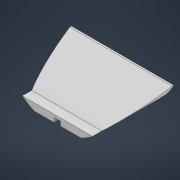
# Autodesk Inventor part: SlopeFloor
Saved by Autodesk Inventor 2021 (Build 250183000, 183)
## iProperties
Created: 2021-01-31
Part Number: SlopeFloor
Material: Generic
Document SubType Name: Modeling
Designer: argon
Density: 1 g/cm^3
Appearance: Light Gray
Author: argon
Autodesk Inventor part; units mm, degrees
ref_plane "YZ Plane" through (0, 0, 0) normal (1, 0, 0) x (0, 1, 0)
ref_plane "XZ Plane" through (0, 0, 0) normal (0, 1, 0) x (-1, 0, 0)
ref_plane "XY Plane" through (0, 0, 0) normal (0, 0, 1) x (1, 0, 0)
sketch "Sketch1" plane through (0, 0, 0) normal (0, 0, 1) x (1, 0, 0)
  circle A0 centre (0, 0) radius 1750
  line L0 (-1569.0363, -775) -> (1569.0363, -775)
  line L1 (-64, -1498) -> (64, -1498)
  line L2 (64, -1498) -> (64, -1600)
  line L3 (64, -1600) -> (-64, -1600)
  line L4 (-64, -1600) -> (-64, -1498)
  line L5 (-64, -1498) -> (64, -1600) construction
  line L6 (64, -1498) -> (-64, -1600) construction
  line L7 (97, -1633) -> (97, -1465)
  line L8 (97, -1465) -> (-97, -1465)
  line L9 (-97, -1465) -> (-97, -1633)
  line L10 (-97, -1633) -> (97, -1465) construction
  line L11 (97, -1633) -> (-97, -1465) construction
  line L12 (-708.8723, -1600) -> (708.8723, -1600)
  point P0 (0, -1549)
  point P1 (0, -1549)
  point P2 (97, -1600)
  point P3 (-97, -1600)
  dimension "d10" = 3500
  dimension "d12" = 33
  dimension "d13" = 33
  dimension "d14" = 102
  dimension "d15" = 128
  dimension "d16" = 1600
  dimension "d17" = 825
  constraints: 26 end point, 5 midpoint, 4 point on circle, 3 horizontal, 3 parallel, 1 centre point, 1 coincident, 1 collinear, 1 perpendicular, 1 vertical alignment
  measures "d10" diameter of A0
  measures "d12" distance between parallel lines of L2 L7
  measures "d13" distance between parallel lines of L1 L8
  measures "d14" distance of L2.start L2.end
  measures "d15" distance of L4.end L2.start
  measures "d16" distance from line of L3 point (0, 0)
  measures "d17" distance between parallel lines of L12 L0
extrude "Extrusion1" add sketch "Sketch1" along normal blind 2000 contours L0 A0 L12 L7 L8 L9
sketch "Sketch3" plane through (0, 0, 2000) normal (0, 0, 1) x (1, 0, 0)
  arc A0 (-1569.0363, -775) -> (-708.8723, -1600) centre (0, 0) ccw projected
  line L0 (-708.8723, -1600) -> (-97, -1600) projected
  line L1 (-97, -1600) -> (-97, -1465) projected
  line L2 (-97, -1465) -> (97, -1465) projected
  line L3 (97, -1600) -> (708.8723, -1600) projected
  arc A1 (708.8723, -1600) -> (1569.0363, -775) centre (0, 0) ccw projected
  arc A2 (-1569.0363, -775) -> (-708.8723, -1600) centre (0, 0) ccw projected
  arc A3 (708.8723, -1600) -> (1569.0363, -775) centre (0, 0) ccw projected
  line L4 (-1569.0363, -775) -> (1569.0363, -775)
  line L5 (-1076.1505, -1380) -> (1076.1505, -1380)
  dimension "d35" = 605
  constraints: 4 end point, 2 horizontal, 2 point on circle
  measures "d35" distance between parallel lines of L5 L4
extrude "Extrusion3" cut sketch "Sketch3" against normal blind 1950
chamfer "Chamfer1" distance 605 angle 70 1 edges at (0, -1380, 50) measured on face at (-341.0533, -1009.7104, 50)
body "Solid1"
